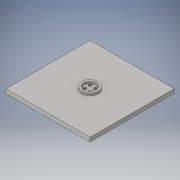
# Autodesk Inventor part: Part1
Saved by Autodesk Inventor 2016 (Build 200138000, 138)
## iProperties
Created: 2016-03-23
Part Number: Part1
Material: Generic
Document SubType Name: Modeling
Designer: Dhivya Sukumar
Density: 1 g/cm^3
Appearance: Default
Author: Dhivya Sukumar
Autodesk Inventor part; units mm, degrees
ref_plane "YZ Plane" through (0, 0, 0) normal (1, 0, 0) x (0, 1, 0)
ref_plane "XZ Plane" through (0, 0, 0) normal (0, 1, 0) x (-1, 0, 0)
ref_plane "XY Plane" through (0, 0, 0) normal (0, 0, 1) x (1, 0, 0)
sketch "Sketch1" plane through (0, 0, 0) normal (0, 1, 0) x (-1, 0, 0)
  line L0 (0, 0) -> (-127, 0)
  line L1 (-127, 0) -> (-127, -127)
  line L2 (-127, -127) -> (0, -127)
  line L3 (0, -127) -> (0, 0)
  dimension "d0" = 127
  dimension "d1" = 127
  constraints: 8 end point, 2 parallel, 1 horizontal, 1 perpendicular
  measures "d0" distance of L2.end L1.end
  measures "d1" distance of L1.end L0.end
extrude "Extrusion1" add sketch "Sketch1" along normal blind 6.35
sketch "Sketch2" plane through (0, 6.35, 0) normal (0, 1, 0) x (1, 0, 0)
  line L0 (0, 0) -> (127, 0) projected
  line L1 (127, 0) -> (127, 127) projected
  line L2 (56.7828, 56.7828) -> (70.2172, 70.2172)
  line L3 (127, 127) -> (127, 0)
  line L4 (70.2172, 56.7828) -> (56.7828, 70.2172)
  line L5 (0, 127) -> (0, 0) projected
  circle A0 centre (63.5, 63.5) radius 9.4996
  circle A1 centre (63.5, 63.5) radius 12.8477
  constraints: 7 end point, 4 point on circle, 2 centre point, 1 collinear, 1 midpoint, 1 perpendicular
extrude "Extrusion2" add sketch "Sketch2" along normal blind 2.9972
sketch "Sketch3" plane through (63.5, 6.35, -63.5) normal (0, 1, 0) x (1, 0, 0)
  circle A0 centre (0, 0) radius 9.4996 projected
  line L0 (9.4891, 0.446) -> (9.7729, 0.446) construction
  line L1 (-5.8104, 5.9947) -> (-6.6345, 6.7989)
  circle A1 centre (3.7745, 4.4415) radius 2.413
  circle A2 centre (4.4123, -3.9814) radius 2.413
  circle A3 centre (-4.3831, -3.9179) radius 2.413
  circle A4 centre (-4.0835, 4.3094) radius 2.413
  line L2 (6.1393, -5.6667) -> (6.9589, -6.4665)
  line L3 (5.4598, 6.1684) -> (6.3421, 7.0725)
  line L4 (-6.9155, -6.5129) -> (-6.0684, -5.6448)
  line L5 (6.9589, -6.4665) -> (6.1393, -5.6667)
  point P0 (-63.5, -63.5)
  constraints: 12 end point, 5 point on circle, 1 collinear, 1 horizontal, 1 perpendicular, 1 point on line, 12 other
hole "Hole1" at (67.4966, 6.35, -67.8963) direction (0, -1, 0) diameter 4.826 end through all
hole "Hole2" at (59.2369, 6.35, -68.1627) direction (0, -1, 0) diameter 4.826 end through all
hole "Hole3" at (59.2369, 6.35, -59.903) direction (0, -1, 0) diameter 4.826 end through all
hole "Hole4" at (67.9123, 6.35, -59.5186) direction (0, -1, 0) diameter 4.826 end through all
body "Solid1"
